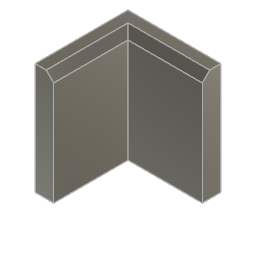
corner v2 (Autodesk Fusion 360 design; units mm, degrees)
Autodesk Fusion 360 part; units mm, degrees
sketch "Sketch1" plane through (0, 0, 0) normal (0, 0, 1) x (1, 0, 0)
  line L0 (0, 0) -> (0, 25)
  line L1 (0, 25) -> (25, 25)
  line L2 (25, 25) -> (25, 20)
  line L3 (0, 0) -> (5, 0)
  line L4 (5, 0) -> (5, 20)
  line L5 (5, 20) -> (25, 20)
  dimension "d5" = 25
  dimension "d6" = 25
  dimension "d7" = 5
  dimension "d8" = 5
  constraint coincident L0.start L3.start
  constraint vertical L0
  constraint perpendicular L0 L1
  constraint perpendicular L1 L2
  constraint perpendicular L0 L3
  constraint perpendicular L3 L4
  measures "d5" distance of L0.start L0.end
  measures "d6" distance of L0.end L1.end
  measures "d7" distance of L1.end L2.end
  measures "d8" distance of L0.start L3.end
extrude "Extrude1" add sketch "Sketch1" along normal blind 30
chamfer "Chamfer1" distance 2 angle 45 1 edges at (5, 10, 30)
chamfer "Chamfer2" distance 2 angle 45 1 edges at (14, 20, 30)
sketch "Sketch2" plane through (0, 0, 0) normal (0, 0, -1) x (1, 0, 0)
  line L0 (5, 0) -> (0, 0)
  line L1 (0, 0) -> (0, -25)
  line L2 (0, -25) -> (25, -25)
  line L3 (25, -25) -> (25, -20)
  line L4 (25, -20) -> (5, -20)
  line L5 (5, -20) -> (5, 0)
  line L6 (1.5, -2) -> (3.5, -2)
  line L7 (1.5, -21.5) -> (1.5, -23.5)
  line L8 (23, -21.5) -> (23, -23.5)
  line L9 (3.5, -2) -> (3.5, -21.5)
  line L10 (1.5, -2) -> (1.5, -21.5)
  line L11 (23, -21.5) -> (3.5, -21.5)
  line L12 (23, -23.5) -> (1.5, -23.5)
  dimension "d13" = 2
  dimension "d14" = 1.5
  dimension "d18" = 1.5
  dimension "d19" = 2
  dimension "d20" = 2
  dimension "d21" = 2
  constraint perpendicular L1 L6
  constraint perpendicular L0 L9
  constraint perpendicular L6 L10
  constraint perpendicular L9 L11
  measures "d13" distance of L6.start L6.end
  measures "d14" distance of L1 L6.start
  measures "d18" distance of L2 L8.end
  measures "d19" distance of L8.start L8.end
  measures "d20" distance of L3 L8
  measures "d21" distance of L0 L6
extrude "Extrude2" cut sketch "Sketch2" against normal blind 22 contours L6 L7 L8 L9 L10 L11 L12
